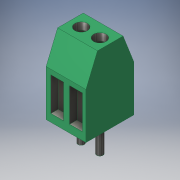
# Autodesk Inventor part: Screw_Terminal_3Pos
Saved by Autodesk Inventor 2016 (Build 200138000, 138)
## iProperties
Created: 2016-09-29
Part Number: Screw_Terminal_3Pos
Material: Generic
Document SubType Name: Modeling
Designer: jfixelle
Density: 1 g/cm^3
Appearance: Smooth - Dark Sea Green
Author: jfixelle
Autodesk Inventor part; units mm, degrees
ref_plane "YZ Plane" through (0, 0, 0) normal (1, 0, 0) x (0, 1, 0)
ref_plane "XZ Plane" through (0, 0, 0) normal (0, 1, 0) x (-1, 0, 0)
ref_plane "XY Plane" through (0, 0, 0) normal (0, 0, 1) x (1, 0, 0)
sketch "Sketch1" plane through (0, 0, 0) normal (1, 0, 0) x (0, 1, 0)
  line L0 (0, 3.25) -> (10, 3.25)
  line L1 (10, 3.25) -> (10, -3.25)
  line L2 (10, -3.25) -> (0, -3.25)
  line L3 (0, -3.25) -> (0, 3.25)
  line L4 (10, 1.6898) -> (6.2365, 3.25)
  line L5 (10, -1.7859) -> (6.2365, -3.25)
  point P0 (0, 0)
  dimension "d0" = 10
  dimension "d1" = 6.5
  dimension "d2" = 3.25
  dimension "d3" = 0
  constraints: 12 end point, 4 point on line, 2 parallel, 1 horizontal, 1 perpendicular
  measures "d0" distance of L1.end L2.end
  measures "d1" distance of L0.end L1.end
  measures "d2" distance from line of point (0, 0) L0
  measures "d3" distance from line of point (0, 0) L3
extrude "Extrusion1" add sketch "Sketch1" along normal blind 3.9 and the other way blind 1.5 contours L0 L4 L1 L5 L2 L3
sketch "Sketch2" plane through (-1.5, 0, -3.25) normal (0, -1, 0) x (1, 0, 0)
  circle A0 centre (1.5, 3.25) radius 0.425
  line L0 (0, 0) -> (0, 6.5) projected
  dimension "d7" = 0.85
  dimension "d12" = 1.5
  constraints: 1 centre point
  measures "d7" diameter of A0
  measures "d12" distance from line of L0 A0.centre
extrude "Extrusion2" add sketch "Sketch2" along normal blind 3.6
sketch "Sketch3" plane through (-1.5, 10, 1.6898) normal (0, 1, 0) x (1, 0, 0)
  circle A0 centre (1.5, 1.6898) radius 0.8517
  constraints: 1 centre point, 1 coincident
extrude "Extrusion3" cut sketch "Sketch3" against normal blind 1
sketch "Sketch4" plane through (-1.5, 0, 3.25) normal (0, 0, 1) x (1, 0, 0)
  line L0 (0.648, 5.5866) -> (2.3749, 5.5866)
  line L1 (2.3749, 5.5866) -> (2.3749, 1.0456)
  line L2 (2.3749, 1.0456) -> (0.648, 1.0456)
  line L3 (0.648, 1.0456) -> (0.648, 5.5866)
  point P0 (1.5, 0)
  constraints: 8 end point, 2 parallel, 1 horizontal, 1 perpendicular
extrude "Extrusion4" cut sketch "Sketch4" against normal blind 1
pattern_linear "Rectangular Pattern1" count 2 spacing 2.54 along (1, 0, 0) of "Extrusion4", "Extrusion3", "Extrusion2"
body "Solid1"
